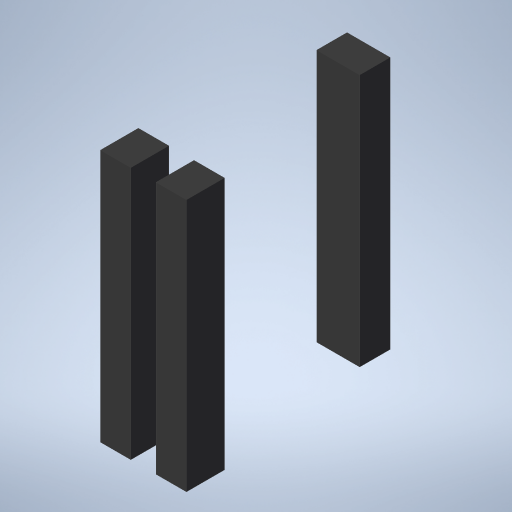
# Autodesk Inventor part: hv_trans_footprint
Saved by Autodesk Inventor 2023.2 (Build 272271000, 271)
## iProperties
Created: 2023-07-25
Part Number: hv_trans_footprint
Material: Generic
Document SubType Name: Modeling
Designer: yiako
Density: 1 g/cm^3
Appearance: Default
Author: yiako
Autodesk Inventor part; units mm, degrees
ref_plane "YZ Plane" through (0, 0, 0) normal (1, 0, 0) x (0, 1, 0)
ref_plane "XZ Plane" through (0, 0, 0) normal (0, 1, 0) x (-1, 0, 0)
ref_plane "XY Plane" through (0, 0, 0) normal (0, 0, 1) x (1, 0, 0)
sketch "Sketch1" plane through (0, 0, 0) normal (0, 1, 0) x (-1, 0, 0)
  line L0 (0, 0) -> (1.2, 0)
  line L1 (1.2, 0) -> (1.2, -1.5)
  line L2 (1.2, -1.5) -> (0, -1.5)
  line L3 (0, -1.5) -> (0, 0)
  line L4 (3.4, 0) -> (2.2, 0)
  line L5 (2.2, 0) -> (2.2, -1.5)
  line L6 (2.2, -1.5) -> (3.4, -1.5)
  line L7 (3.4, -1.5) -> (3.4, 0)
  line L8 (0.85, -7.7) -> (2.55, -7.7)
  line L9 (2.55, -7.7) -> (2.55, -8.9)
  line L10 (2.55, -8.9) -> (0.85, -8.9)
  line L11 (0.85, -8.9) -> (0.85, -7.7)
  point P0 (1.2, -0.75)
  dimension "d0" = 1.2
  dimension "d1" = 1.5
  dimension "d5" = 1.2
  dimension "d6" = 1.5
  dimension "d7" = 1
  dimension "d8" = 1.7
  dimension "d9" = 1.2
  dimension "d10" = 6.2
  dimension "d11" = 0.85
  constraints: 24 end point, 6 parallel, 3 horizontal, 3 perpendicular, 1 midpoint
  measures "d0" distance of L1.end L2.end
  measures "d1" distance of L0.end L1.end
  measures "d5" distance of L6.end L5.end
  measures "d6" distance of L5.end L4.end
  measures "d7" distance between parallel lines of L1 L5
  measures "d8" distance of L9.end L10.end
  measures "d9" distance of L8.end L9.end
  measures "d10" distance between parallel lines of L8 L2
  measures "d11" distance between parallel lines of L3 L11
extrude "Extrusion1" add sketch "Sketch1" along normal blind 10
body "Solid1"
